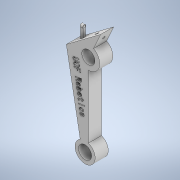
# Autodesk Inventor part: legV.1
Saved by Autodesk Inventor 2022 (Build 260153000, 153)
## iProperties
Created: 2022-01-23
Part Number: legV.1
Material: Generic
Document SubType Name: Modeling
Designer: money
Density: 1 g/cm^3
Appearance: Default
Author: money
Autodesk Inventor part; units mm, degrees
note: some values were not read from the file. Chosen so that the rebuilt part matches the saved one: sketch regions of "Extrusion1".
ref_plane "YZ Plane" through (0, 0, 0) normal (1, 0, 0) x (0, 1, 0)
ref_plane "XZ Plane" through (0, 0, 0) normal (0, 1, 0) x (-1, 0, 0)
ref_plane "XY Plane" through (0, 0, 0) normal (0, 0, 1) x (1, 0, 0)
sketch "Sketch1" plane through (0, 0, 0) normal (0, 0, 1) x (1, 0, 0)
  line L0 (25.584, 74.5203) -> (-8.8379, 48.7039)
  line L1 (25.584, 74.5203) -> (18.6122, 58.7142)
  arc A0 (13.3627, 37.1685) -> (18.6122, 58.7142) centre (13.3627, 48.5808) ccw
  circle A1 centre (13.3627, 48.5808) radius 6.604
  arc A2 (5.1377, -27.1634) -> (13.3627, -26.4893) centre (10.0086, -36.0797) ccw
  line L2 (-8.8379, 48.7039) -> (5.1377, -27.1634)
  line L3 (14.1717, -76.2055) -> (14.4802, -77.8797)
  line L4 (13.3627, 37.1685) -> (13.3627, -26.4893)
  circle A3 centre (10.0086, -36.0797) radius 6.604
  line L5 (3.7654, 42.7726) -> (3.9013, 41.8845)
  line L6 (3.9013, 41.8845) -> (-0.6634, 41.186)
  spline S0 degree 2 poles (-0.6634, 41.186) (-1.1355, 41.1137) (-1.3021, 40.8917) knots 0 0 0 1 1 1
  spline S1 degree 2 poles (-1.3021, 40.8917) (-1.4682, 40.6657) (-1.4063, 40.2616) knots 0 0 0 1 1 1
  line L7 (-1.4063, 40.2616) -> (-1.4014, 40.2296)
  spline S2 degree 2 poles (-1.4014, 40.2296) (-1.3439, 39.8536) (-1.1179, 39.6875) knots 0 0 0 1 1 1
  spline S3 degree 2 poles (-1.1179, 39.6875) (-0.8549, 39.4944) (-0.4149, 39.5617) knots 0 0 0 1 1 1
  line L8 (-0.4149, 39.5617) -> (4.1498, 40.2602)
  line L9 (4.1498, 40.2602) -> (4.2851, 39.3761)
  line L10 (4.2851, 39.3761) -> (-0.2796, 38.6776)
  spline S4 degree 2 poles (-0.2796, 38.6776) (-1.1317, 38.5472) (-1.6997, 38.968) knots 0 0 0 1 1 1
  spline S5 degree 2 poles (-1.6997, 38.968) (-2.1241, 39.2797) (-2.2496, 40.0998) knots 0 0 0 1 1 1
  line L11 (-2.2496, 40.0998) -> (-2.2545, 40.1318)
  spline S6 degree 2 poles (-2.2545, 40.1318) (-2.38, 40.952) (-2.0682, 41.3763) knots 0 0 0 1 1 1
  spline S7 degree 2 poles (-2.0682, 41.3763) (-1.6514, 41.9437) (-0.7993, 42.0741) knots 0 0 0 1 1 1
  line L12 (-0.7993, 42.0741) -> (3.7654, 42.7726)
  spline S8 degree 2 poles (1.1719, 34.5434) (-0.371, 34.4056) (-0.9753, 34.8495) knots 0 0 0 1 1 1
  spline S9 degree 2 poles (-0.9753, 34.8495) (-1.5058, 35.2391) (-1.6031, 35.8752) knots 0 0 0 1 1 1
  spline S10 degree 2 poles (-1.6031, 35.8752) (-1.6992, 36.5033) (-1.3102, 37.0378) knots 0 0 0 1 1 1
  spline S11 degree 2 poles (-1.3102, 37.0378) (-0.6257, 37.9696) (1.0706, 38.2291) knots 0 0 0 1 1 1
  spline S12 degree 2 poles (1.0706, 38.2291) (3.0509, 38.5321) (4.0524, 37.7929) knots 0 0 0 1 1 1
  spline S13 degree 2 poles (4.0524, 37.7929) (4.5875, 37.3998) (4.6787, 36.8037) knots 0 0 0 1 1 1
  spline S14 degree 2 poles (4.6787, 36.8037) (4.7755, 36.1716) (4.4637, 35.7472) knots 0 0 0 1 1 1
  spline S15 degree 2 poles (4.4637, 35.7472) (3.8843, 34.9585) (2.6392, 34.8007) knots 0 0 0 1 1 1
  line L13 (2.6392, 34.8007) -> (2.5088, 35.6528)
  spline S16 degree 2 poles (2.5088, 35.6528) (3.5521, 35.8452) (3.8265, 36.2188) knots 0 0 0 1 1 1
  spline S17 degree 2 poles (3.8265, 36.2188) (3.9655, 36.408) (3.9226, 36.688) knots 0 0 0 1 1 1
  spline S18 degree 2 poles (3.9226, 36.688) (3.8853, 36.9321) (3.6586, 37.1021) knots 0 0 0 1 1 1
  spline S19 degree 2 poles (3.6586, 37.1021) (2.9627, 37.6097) (1.2705, 37.3508) knots 0 0 0 1 1 1
  spline S20 degree 2 poles (1.2705, 37.3508) (-0.2057, 37.1249) (-0.6361, 36.5391) knots 0 0 0 1 1 1
  spline S21 degree 2 poles (-0.6361, 36.5391) (-0.8292, 36.2761) (-0.787, 36.0001) knots 0 0 0 1 1 1
  spline S22 degree 2 poles (-0.787, 36.0001) (-0.7484, 35.7481) (-0.4861, 35.5589) knots 0 0 0 1 1 1
  spline S23 degree 2 poles (-0.4861, 35.5589) (-0.1494, 35.3116) (1.0323, 35.4555) knots 0 0 0 1 1 1
  line L14 (1.0323, 35.4555) -> (1.1719, 34.5434)
  line L15 (-1.2517, 33.5789) -> (5.0252, 34.5394)
  line L16 (5.0252, 34.5394) -> (5.5548, 31.0789)
  line L17 (5.5548, 31.0789) -> (4.7986, 30.9632)
  line L18 (4.7986, 30.9632) -> (4.4044, 33.5395)
  line L19 (4.4044, 33.5395) -> (2.5241, 33.2518)
  line L20 (2.5241, 33.2518) -> (2.8223, 31.3035)
  line L21 (2.8223, 31.3035) -> (2.0661, 31.1878)
  line L22 (2.0661, 31.1878) -> (1.768, 33.1361)
  line L23 (1.768, 33.1361) -> (-1.1164, 32.6947)
  line L24 (-1.1164, 32.6947) -> (-1.2517, 33.5789)
  spline S24 degree 2 poles (6.5275, 24.7219) (6.653, 23.9018) (6.2097, 23.2935) knots 0 0 0 1 1 1
  spline S25 degree 2 poles (6.2097, 23.2935) (5.8438, 22.7953) (5.0597, 22.6754) knots 0 0 0 1 1 1
  spline S26 degree 2 poles (5.0597, 22.6754) (4.3396, 22.5652) (3.814, 22.9228) knots 0 0 0 1 1 1
  spline S27 degree 2 poles (3.814, 22.9228) (3.432, 23.1714) (3.3227, 23.4045) knots 0 0 0 1 1 1
  line L25 (3.3227, 23.4045) -> (0.5469, 21.8251)
  line L26 (0.5469, 21.8251) -> (0.4104, 22.7173)
  line L27 (0.4104, 22.7173) -> (3.0713, 24.2176)
  line L28 (3.0713, 24.2176) -> (2.9587, 24.9537)
  line L29 (2.9587, 24.9537) -> (0.1343, 24.5215)
  line L30 (0.1343, 24.5215) -> (-0.0016, 25.4097)
  line L31 (-0.0016, 25.4097) -> (6.2753, 26.3702)
  line L32 (6.2753, 26.3702) -> (6.5275, 24.7219)
  spline S28 degree 2 poles (3.8409, 24.2453) (3.8936, 23.9012) (4.1888, 23.6844) knots 0 0 0 1 1 1
  spline S29 degree 2 poles (4.1888, 23.6844) (4.4517, 23.4912) (4.9238, 23.5635) knots 0 0 0 1 1 1
  spline S30 degree 2 poles (4.9238, 23.5635) (5.3558, 23.6296) (5.5767, 23.9254) knots 0 0 0 1 1 1
  spline S31 degree 2 poles (5.5767, 23.9254) (5.824, 24.2622) (5.7475, 24.7622) knots 0 0 0 1 1 1
  line L33 (5.7475, 24.7622) -> (5.6551, 25.3663)
  line L34 (5.6551, 25.3663) -> (3.7148, 25.0694)
  line L35 (3.7148, 25.0694) -> (3.8409, 24.2453)
  spline S32 degree 2 poles (4.6294, 21.4467) (5.2337, 21.0029) (5.3445, 20.2788) knots 0 0 0 1 1 1
  spline S33 degree 2 poles (5.3445, 20.2788) (5.451, 19.5826) (5.0072, 18.9784) knots 0 0 0 1 1 1
  spline S34 degree 2 poles (5.0072, 18.9784) (4.5599, 18.3695) (3.3677, 18.1871) knots 0 0 0 1 1 1
  spline S35 degree 2 poles (3.3677, 18.1871) (2.2075, 18.0095) (1.5986, 18.4568) knots 0 0 0 1 1 1
  spline S36 degree 2 poles (1.5986, 18.4568) (0.9944, 18.9007) (0.8879, 19.5968) knots 0 0 0 1 1 1
  spline S37 degree 2 poles (0.8879, 19.5968) (0.777, 20.3209) (1.2209, 20.9252) knots 0 0 0 1 1 1
  spline S38 degree 2 poles (1.2209, 20.9252) (1.6642, 21.5334) (2.8284, 21.7116) knots 0 0 0 1 1 1
  spline S39 degree 2 poles (2.8284, 21.7116) (4.0246, 21.8946) (4.6294, 21.4467) knots 0 0 0 1 1 1
  spline S40 degree 2 poles (4.6204, 20.1679) (4.5684, 20.508) (4.2685, 20.7282) knots 0 0 0 1 1 1
  spline S41 degree 2 poles (4.2685, 20.7282) (3.8995, 20.9993) (2.9594, 20.8555) knots 0 0 0 1 1 1
  spline S42 degree 2 poles (2.9594, 20.8555) (2.0512, 20.7165) (1.7802, 20.3475) knots 0 0 0 1 1 1
  spline S43 degree 2 poles (1.7802, 20.3475) (1.5599, 20.0476) (1.612, 19.7076) knots 0 0 0 1 1 1
  spline S44 degree 2 poles (1.612, 19.7076) (1.6597, 19.3955) (1.9595, 19.1753) knots 0 0 0 1 1 1
  spline S45 degree 2 poles (1.9595, 19.1753) (2.3286, 18.9042) (3.2367, 19.0432) knots 0 0 0 1 1 1
  spline S46 degree 2 poles (3.2367, 19.0432) (4.1728, 19.1864) (4.4479, 19.5561) knots 0 0 0 1 1 1
  spline S47 degree 2 poles (4.4479, 19.5561) (4.6682, 19.8559) (4.6204, 20.1679) knots 0 0 0 1 1 1
  spline S48 degree 2 poles (5.148, 16.961) (5.8936, 16.6902) (6.0008, 15.9901) knots 0 0 0 1 1 1
  spline S49 degree 2 poles (6.0008, 15.9901) (6.0828, 15.454) (5.744, 14.9928) knots 0 0 0 1 1 1
  spline S50 degree 2 poles (5.744, 14.9928) (5.2967, 14.3839) (4.0765, 14.1972) knots 0 0 0 1 1 1
  spline S51 degree 2 poles (4.0765, 14.1972) (2.7883, 14) (2.1794, 14.4473) knots 0 0 0 1 1 1
  spline S52 degree 2 poles (2.1794, 14.4473) (1.6121, 14.8641) (1.53, 15.4002) knots 0 0 0 1 1 1
  spline S53 degree 2 poles (1.53, 15.4002) (1.4327, 16.0363) (1.9115, 16.4657) knots 0 0 0 1 1 1
  line L36 (1.9115, 16.4657) -> (1.3794, 16.3843)
  line L37 (1.3794, 16.3843) -> (1.2582, 17.1764)
  line L38 (1.2582, 17.1764) -> (7.5352, 18.1369)
  line L39 (7.5352, 18.1369) -> (7.6564, 17.3448)
  line L40 (7.6564, 17.3448) -> (5.148, 16.961)
  spline S54 degree 2 poles (3.4997, 16.7088) (2.6196, 16.5741) (2.3756, 16.242) knots 0 0 0 1 1 1
  spline S55 degree 2 poles (2.3756, 16.242) (2.1554, 15.9421) (2.1976, 15.6661) knots 0 0 0 1 1 1
  spline S56 degree 2 poles (2.1976, 15.6661) (2.2503, 15.322) (2.4763, 15.156) knots 0 0 0 1 1 1
  spline S57 degree 2 poles (2.4763, 15.156) (2.9191, 14.8307) (3.8913, 14.9795) knots 0 0 0 1 1 1
  spline S58 degree 2 poles (3.8913, 14.9795) (4.8274, 15.1227) (5.1296, 15.5293) knots 0 0 0 1 1 1
  spline S59 degree 2 poles (5.1296, 15.5293) (5.2956, 15.7553) (5.2479, 16.0673) knots 0 0 0 1 1 1
  spline S60 degree 2 poles (5.2479, 16.0673) (5.2008, 16.3754) (4.864, 16.6227) knots 0 0 0 1 1 1
  spline S61 degree 2 poles (4.864, 16.6227) (4.5319, 16.8667) (3.4997, 16.7088) knots 0 0 0 1 1 1
  spline S62 degree 2 poles (5.8844, 13.2455) (6.4887, 12.8016) (6.5995, 12.0775) knots 0 0 0 1 1 1
  spline S63 degree 2 poles (6.5995, 12.0775) (6.706, 11.3814) (6.2621, 10.7772) knots 0 0 0 1 1 1
  spline S64 degree 2 poles (6.2621, 10.7772) (5.8148, 10.1683) (4.6227, 9.9858) knots 0 0 0 1 1 1
  spline S65 degree 2 poles (4.6227, 9.9858) (3.4625, 9.8083) (2.8536, 10.2556) knots 0 0 0 1 1 1
  spline S66 degree 2 poles (2.8536, 10.2556) (2.2493, 10.6995) (2.1428, 11.3956) knots 0 0 0 1 1 1
  spline S67 degree 2 poles (2.1428, 11.3956) (2.032, 12.1197) (2.4759, 12.7239) knots 0 0 0 1 1 1
  spline S68 degree 2 poles (2.4759, 12.7239) (2.9192, 13.3322) (4.0833, 13.5104) knots 0 0 0 1 1 1
  spline S69 degree 2 poles (4.0833, 13.5104) (5.2795, 13.6934) (5.8844, 13.2455) knots 0 0 0 1 1 1
  spline S70 degree 2 poles (5.8754, 11.9667) (5.8233, 12.3068) (5.5235, 12.527) knots 0 0 0 1 1 1
  spline S71 degree 2 poles (5.5235, 12.527) (5.1545, 12.7981) (4.2143, 12.6542) knots 0 0 0 1 1 1
  spline S72 degree 2 poles (4.2143, 12.6542) (3.3062, 12.5153) (3.0351, 12.1462) knots 0 0 0 1 1 1
  spline S73 degree 2 poles (3.0351, 12.1462) (2.8149, 11.8464) (2.8669, 11.5064) knots 0 0 0 1 1 1
  spline S74 degree 2 poles (2.8669, 11.5064) (2.9147, 11.1943) (3.2145, 10.9741) knots 0 0 0 1 1 1
  spline S75 degree 2 poles (3.2145, 10.9741) (3.5835, 10.703) (4.4917, 10.842) knots 0 0 0 1 1 1
  spline S76 degree 2 poles (4.4917, 10.842) (5.4278, 10.9852) (5.7029, 11.3548) knots 0 0 0 1 1 1
  spline S77 degree 2 poles (5.7029, 11.3548) (5.9231, 11.6547) (5.8754, 11.9667) knots 0 0 0 1 1 1
  line L41 (6.4487, 8.648) -> (6.2951, 9.6522)
  line L42 (6.2951, 9.6522) -> (6.9552, 9.7532)
  line L43 (6.9552, 9.7532) -> (7.1088, 8.749)
  line L44 (7.1088, 8.749) -> (8.489, 8.9602)
  line L45 (8.489, 8.9602) -> (8.6102, 8.1681)
  line L46 (8.6102, 8.1681) -> (7.23, 7.9569)
  line L47 (7.23, 7.9569) -> (7.4461, 6.5447)
  line L48 (7.4461, 6.5447) -> (6.786, 6.4437)
  line L49 (6.786, 6.4437) -> (6.5699, 7.8559)
  line L50 (6.5699, 7.8559) -> (3.7935, 7.4311)
  spline S78 degree 2 poles (3.7935, 7.4311) (3.5295, 7.3907) (3.5937, 6.9706) knots 0 0 0 1 1 1
  spline S79 degree 2 poles (3.5937, 6.9706) (3.6727, 6.4545) (4.0224, 5.8284) knots 0 0 0 1 1 1
  line L51 (4.0224, 5.8284) -> (3.2223, 5.7059)
  spline S80 degree 2 poles (3.2223, 5.7059) (2.8878, 6.5268) (2.8229, 6.9509) knots 0 0 0 1 1 1
  spline S81 degree 2 poles (2.8229, 6.9509) (2.6521, 8.0671) (3.5483, 8.2042) knots 0 0 0 1 1 1
  line L52 (3.5483, 8.2042) -> (6.4487, 8.648)
  line L53 (3.4541, 2.8263) -> (3.3329, 3.6184)
  line L54 (3.3329, 3.6184) -> (7.7896, 4.3004)
  line L55 (7.7896, 4.3004) -> (7.9108, 3.5083)
  line L56 (7.9108, 3.5083) -> (3.4541, 2.8263)
  line L57 (9.731, 3.7868) -> (8.7549, 3.6374)
  line L58 (8.7549, 3.6374) -> (8.6337, 4.4295)
  line L59 (8.6337, 4.4295) -> (9.6098, 4.5789)
  line L60 (9.6098, 4.5789) -> (9.731, 3.7868)
  spline S82 degree 2 poles (6.9635, -1.2182) (7.4932, -1.0675) (7.6666, -0.8363) knots 0 0 0 1 1 1
  spline S83 degree 2 poles (7.6666, -0.8363) (7.8056, -0.6472) (7.7676, -0.3991) knots 0 0 0 1 1 1
  spline S84 degree 2 poles (7.7676, -0.3991) (7.7205, -0.0911) (7.4206, 0.1292) knots 0 0 0 1 1 1
  spline S85 degree 2 poles (7.4206, 0.1292) (7.0147, 0.4274) (6.0146, 0.2743) knots 0 0 0 1 1 1
  spline S86 degree 2 poles (6.0146, 0.2743) (5.1984, 0.1494) (4.9274, -0.2196) knots 0 0 0 1 1 1
  spline S87 degree 2 poles (4.9274, -0.2196) (4.7065, -0.5154) (4.7543, -0.8275) knots 0 0 0 1 1 1
  spline S88 degree 2 poles (4.7543, -0.8275) (4.7971, -1.1075) (5.06, -1.3007) knots 0 0 0 1 1 1
  spline S89 degree 2 poles (5.06, -1.3007) (5.3922, -1.5446) (6.128, -1.4034) knots 0 0 0 1 1 1
  line L61 (6.128, -1.4034) -> (6.2627, -2.2835)
  spline S90 degree 2 poles (6.2627, -2.2835) (5.276, -2.4713) (4.6671, -2.024) knots 0 0 0 1 1 1
  spline S91 degree 2 poles (4.6671, -2.024) (4.1367, -1.6344) (4.0302, -0.9383) knots 0 0 0 1 1 1
  spline S92 degree 2 poles (4.0302, -0.9383) (3.9236, -0.2422) (4.3675, 0.3621) knots 0 0 0 1 1 1
  spline S93 degree 2 poles (4.3675, 0.3621) (4.8385, 1.0033) (5.8787, 1.1624) knots 0 0 0 1 1 1
  spline S94 degree 2 poles (5.8787, 1.1624) (7.0708, 1.3449) (7.7858, 0.8197) knots 0 0 0 1 1 1
  spline S95 degree 2 poles (7.7858, 0.8197) (8.3901, 0.3758) (8.4917, -0.2883) knots 0 0 0 1 1 1
  spline S96 degree 2 poles (8.4917, -0.2883) (8.5927, -0.9484) (8.2539, -1.4097) knots 0 0 0 1 1 1
  spline S97 degree 2 poles (8.2539, -1.4097) (7.8919, -1.9073) (7.0933, -2.0663) knots 0 0 0 1 1 1
  line L62 (7.0933, -2.0663) -> (6.9635, -1.2182)
  spline S98 degree 2 poles (7.7644, -5.194) (8.1469, -5.0986) (8.2892, -4.9049) knots 0 0 0 1 1 1
  spline S99 degree 2 poles (8.2892, -4.9049) (8.4282, -4.7158) (8.3853, -4.4357) knots 0 0 0 1 1 1
  spline S100 degree 2 poles (8.3853, -4.4357) (8.3284, -4.0637) (8.1761, -3.9518) knots 0 0 0 1 1 1
  spline S101 degree 2 poles (8.1761, -3.9518) (7.987, -3.8129) (7.799, -3.8417) knots 0 0 0 1 1 1
  spline S102 degree 2 poles (7.799, -3.8417) (7.675, -3.8607) (7.5632, -4.0129) knots 0 0 0 1 1 1
  spline S103 degree 2 poles (7.5632, -4.0129) (7.387, -4.2528) (7.2423, -5.02) knots 0 0 0 1 1 1
  spline S104 degree 2 poles (7.2423, -5.02) (7.1434, -5.6043) (6.9198, -5.9087) knots 0 0 0 1 1 1
  spline S105 degree 2 poles (6.9198, -5.9087) (6.6589, -6.2639) (6.1588, -6.3404) knots 0 0 0 1 1 1
  spline S106 degree 2 poles (6.1588, -6.3404) (5.6867, -6.4127) (5.2946, -6.1247) knots 0 0 0 1 1 1
  spline S107 degree 2 poles (5.2946, -6.1247) (4.7642, -5.735) (4.6527, -5.0069) knots 0 0 0 1 1 1
  spline S108 degree 2 poles (4.6527, -5.0069) (4.5321, -4.2188) (4.867, -3.7581) knots 0 0 0 1 1 1
  spline S109 degree 2 poles (4.867, -3.7581) (5.2335, -3.2639) (6.2306, -3.1441) knots 0 0 0 1 1 1
  line L63 (6.2306, -3.1441) -> (6.3512, -3.9322)
  spline S110 degree 2 poles (6.3512, -3.9322) (5.6151, -4.0449) (5.4762, -4.234) knots 0 0 0 1 1 1
  spline S111 degree 2 poles (5.4762, -4.234) (5.3101, -4.46) (5.372, -4.8641) knots 0 0 0 1 1 1
  spline S112 degree 2 poles (5.372, -4.8641) (5.4344, -5.2721) (5.6604, -5.4382) knots 0 0 0 1 1 1
  spline S113 degree 2 poles (5.6604, -5.4382) (5.8495, -5.5771) (6.0696, -5.5434) knots 0 0 0 1 1 1
  spline S114 degree 2 poles (6.0696, -5.5434) (6.2216, -5.5202) (6.3605, -5.331) knots 0 0 0 1 1 1
  spline S115 degree 2 poles (6.3605, -5.331) (6.5096, -5.1281) (6.6147, -4.5838) knots 0 0 0 1 1 1
  spline S116 degree 2 poles (6.6147, -4.5838) (6.7797, -3.7356) (7.0033, -3.4312) knots 0 0 0 1 1 1
  spline S117 degree 2 poles (7.0033, -3.4312) (7.2608, -3.0806) (7.7049, -3.0127) knots 0 0 0 1 1 1
  spline S118 degree 2 poles (7.7049, -3.0127) (8.145, -2.9453) (8.5693, -3.2571) knots 0 0 0 1 1 1
  spline S119 degree 2 poles (8.5693, -3.2571) (8.9937, -3.5688) (9.1094, -4.3249) knots 0 0 0 1 1 1
  spline S120 degree 2 poles (9.1094, -4.3249) (9.211, -4.989) (8.8722, -5.4503) knots 0 0 0 1 1 1
  spline S121 degree 2 poles (8.8722, -5.4503) (8.5333, -5.9116) (7.8837, -5.9741) knots 0 0 0 1 1 1
  line L64 (7.8837, -5.9741) -> (7.7644, -5.194)
  point P0 (7.4727, 18.545)
  dimension "d2" = 152.4
  dimension "d3" = 10.16
  dimension "d4" = 13.208
  dimension "d5" = 13.208
  constraints: 10 end point, 4 centre point, 4 point on circle, 2 coincident, 1 other
  measures "d2" vertical distance of L3.end L0.start
  measures "d3" radius of A2
  measures "d4" diameter of A3
  measures "d5" diameter of A1
extrude "Extrusion1" add sketch "Sketch1" along normal blind 13.208 contours L1 A0 L4 A2 L2 L0 | L5 L6 S0 S1 L7 S2 S3 L8 L9 L10 S4 S5 L11 S6 S7 L12 | S8 S9 S10 S11 S12 S13 S14 S15 L13 S16 S17 S18 S19 S20 S21 S22 S23 L14 | L15 L16 L17 L18 L19 L20 L21 L22 L23 L24 | S24 S25 S26 S27 L25 L26 L27 L28 L29 L30 L31 L32 | S32 S33 S34 S35 S36 S37 S38 S39 | S48 S49 S50 S51 S52 S53 L36 L37 L38 L39 L40 | S62 S63 S64 S65 S66 S67 S68 S69 | L41 L42 L43 L44 L45 L46 L47 L48 L49 L50 S78 S79 L51 S80 S81 L52 | L53 L54 L55 L56 | L57 L58 L59 L60 | S82 S83 S84 S85 S86 S87 S88 S89 L61 S90 S91 S92 S93 S94 S95 S96 S97 L62 | S98 S99 S100 S101 S102 S103 S104 S105 S106 S107 S108 S109 L63 S110 S111 S112 S113 S114 S115 S116 S117 S118 S119 S120 S121 L64
sketch "Sketch2" plane through (0, 0, 13.208) normal (0, 0, 1) x (1, 0, 0)
  line L0 (3.7654, 42.7726) -> (3.9013, 41.8845)
  line L1 (3.9013, 41.8845) -> (-0.6634, 41.186)
  spline S0 degree 2 poles (-0.6634, 41.186) (-1.1355, 41.1137) (-1.3021, 40.8917) knots 0 0 0 1 1 1
  spline S1 degree 2 poles (-1.3021, 40.8917) (-1.4682, 40.6657) (-1.4063, 40.2616) knots 0 0 0 1 1 1
  line L2 (-1.4063, 40.2616) -> (-1.4014, 40.2296)
  spline S2 degree 2 poles (-1.4014, 40.2296) (-1.3439, 39.8536) (-1.1179, 39.6875) knots 0 0 0 1 1 1
  spline S3 degree 2 poles (-1.1179, 39.6875) (-0.8549, 39.4944) (-0.4149, 39.5617) knots 0 0 0 1 1 1
  line L3 (-0.4149, 39.5617) -> (4.1498, 40.2602)
  line L4 (4.1498, 40.2602) -> (4.2851, 39.3761)
  line L5 (4.2851, 39.3761) -> (-0.2796, 38.6776)
  spline S4 degree 2 poles (-0.2796, 38.6776) (-1.1317, 38.5472) (-1.6997, 38.968) knots 0 0 0 1 1 1
  spline S5 degree 2 poles (-1.6997, 38.968) (-2.1241, 39.2797) (-2.2496, 40.0998) knots 0 0 0 1 1 1
  line L6 (-2.2496, 40.0998) -> (-2.2545, 40.1318)
  spline S6 degree 2 poles (-2.2545, 40.1318) (-2.38, 40.952) (-2.0682, 41.3763) knots 0 0 0 1 1 1
  spline S7 degree 2 poles (-2.0682, 41.3763) (-1.6514, 41.9437) (-0.7993, 42.0741) knots 0 0 0 1 1 1
  line L7 (-0.7993, 42.0741) -> (3.7654, 42.7726)
  spline S8 degree 2 poles (1.1719, 34.5434) (-0.371, 34.4056) (-0.9753, 34.8495) knots 0 0 0 1 1 1
  spline S9 degree 2 poles (-0.9753, 34.8495) (-1.5058, 35.2391) (-1.6031, 35.8752) knots 0 0 0 1 1 1
  spline S10 degree 2 poles (-1.6031, 35.8752) (-1.6992, 36.5033) (-1.3102, 37.0378) knots 0 0 0 1 1 1
  spline S11 degree 2 poles (-1.3102, 37.0378) (-0.6257, 37.9696) (1.0706, 38.2291) knots 0 0 0 1 1 1
  spline S12 degree 2 poles (1.0706, 38.2291) (3.0509, 38.5321) (4.0524, 37.7929) knots 0 0 0 1 1 1
  spline S13 degree 2 poles (4.0524, 37.7929) (4.5875, 37.3998) (4.6787, 36.8037) knots 0 0 0 1 1 1
  spline S14 degree 2 poles (4.6787, 36.8037) (4.7755, 36.1716) (4.4637, 35.7472) knots 0 0 0 1 1 1
  spline S15 degree 2 poles (4.4637, 35.7472) (3.8843, 34.9585) (2.6392, 34.8007) knots 0 0 0 1 1 1
  line L8 (2.6392, 34.8007) -> (2.5088, 35.6528)
  spline S16 degree 2 poles (2.5088, 35.6528) (3.5521, 35.8452) (3.8265, 36.2188) knots 0 0 0 1 1 1
  spline S17 degree 2 poles (3.8265, 36.2188) (3.9655, 36.408) (3.9226, 36.688) knots 0 0 0 1 1 1
  spline S18 degree 2 poles (3.9226, 36.688) (3.8853, 36.9321) (3.6586, 37.1021) knots 0 0 0 1 1 1
  spline S19 degree 2 poles (3.6586, 37.1021) (2.9627, 37.6097) (1.2705, 37.3508) knots 0 0 0 1 1 1
  spline S20 degree 2 poles (1.2705, 37.3508) (-0.2057, 37.1249) (-0.6361, 36.5391) knots 0 0 0 1 1 1
  spline S21 degree 2 poles (-0.6361, 36.5391) (-0.8292, 36.2761) (-0.787, 36.0001) knots 0 0 0 1 1 1
  spline S22 degree 2 poles (-0.787, 36.0001) (-0.7484, 35.7481) (-0.4861, 35.5589) knots 0 0 0 1 1 1
  spline S23 degree 2 poles (-0.4861, 35.5589) (-0.1494, 35.3116) (1.0323, 35.4555) knots 0 0 0 1 1 1
  line L9 (1.0323, 35.4555) -> (1.1719, 34.5434)
  line L10 (-1.2517, 33.5789) -> (5.0252, 34.5394)
  line L11 (5.0252, 34.5394) -> (5.5548, 31.0789)
  line L12 (5.5548, 31.0789) -> (4.7986, 30.9632)
  line L13 (4.7986, 30.9632) -> (4.4044, 33.5395)
  line L14 (4.4044, 33.5395) -> (2.5241, 33.2518)
  line L15 (2.5241, 33.2518) -> (2.8223, 31.3035)
  line L16 (2.8223, 31.3035) -> (2.0661, 31.1878)
  line L17 (2.0661, 31.1878) -> (1.768, 33.1361)
  line L18 (1.768, 33.1361) -> (-1.1164, 32.6947)
  line L19 (-1.1164, 32.6947) -> (-1.2517, 33.5789)
  spline S24 degree 2 poles (6.5275, 24.7219) (6.653, 23.9018) (6.2097, 23.2935) knots 0 0 0 1 1 1
  spline S25 degree 2 poles (6.2097, 23.2935) (5.8438, 22.7953) (5.0597, 22.6754) knots 0 0 0 1 1 1
  spline S26 degree 2 poles (5.0597, 22.6754) (4.3396, 22.5652) (3.814, 22.9228) knots 0 0 0 1 1 1
  spline S27 degree 2 poles (3.814, 22.9228) (3.432, 23.1714) (3.3227, 23.4045) knots 0 0 0 1 1 1
  line L20 (3.3227, 23.4045) -> (0.5469, 21.8251)
  line L21 (0.5469, 21.8251) -> (0.4104, 22.7173)
  line L22 (0.4104, 22.7173) -> (3.0713, 24.2176)
  line L23 (3.0713, 24.2176) -> (2.9587, 24.9537)
  line L24 (2.9587, 24.9537) -> (0.1343, 24.5215)
  line L25 (0.1343, 24.5215) -> (-0.0016, 25.4097)
  line L26 (-0.0016, 25.4097) -> (6.2753, 26.3702)
  line L27 (6.2753, 26.3702) -> (6.5275, 24.7219)
  spline S28 degree 2 poles (3.8409, 24.2453) (3.8936, 23.9012) (4.1888, 23.6844) knots 0 0 0 1 1 1
  spline S29 degree 2 poles (4.1888, 23.6844) (4.4517, 23.4912) (4.9238, 23.5635) knots 0 0 0 1 1 1
  spline S30 degree 2 poles (4.9238, 23.5635) (5.3558, 23.6296) (5.5767, 23.9254) knots 0 0 0 1 1 1
  spline S31 degree 2 poles (5.5767, 23.9254) (5.824, 24.2622) (5.7475, 24.7622) knots 0 0 0 1 1 1
  line L28 (5.7475, 24.7622) -> (5.6551, 25.3663)
  line L29 (5.6551, 25.3663) -> (3.7148, 25.0694)
  line L30 (3.7148, 25.0694) -> (3.8409, 24.2453)
  spline S32 degree 2 poles (4.6294, 21.4467) (5.2337, 21.0029) (5.3445, 20.2788) knots 0 0 0 1 1 1
  spline S33 degree 2 poles (5.3445, 20.2788) (5.451, 19.5826) (5.0072, 18.9784) knots 0 0 0 1 1 1
  spline S34 degree 2 poles (5.0072, 18.9784) (4.5599, 18.3695) (3.3677, 18.1871) knots 0 0 0 1 1 1
  spline S35 degree 2 poles (3.3677, 18.1871) (2.2075, 18.0095) (1.5986, 18.4568) knots 0 0 0 1 1 1
  spline S36 degree 2 poles (1.5986, 18.4568) (0.9944, 18.9007) (0.8879, 19.5968) knots 0 0 0 1 1 1
  spline S37 degree 2 poles (0.8879, 19.5968) (0.777, 20.3209) (1.2209, 20.9252) knots 0 0 0 1 1 1
  spline S38 degree 2 poles (1.2209, 20.9252) (1.6642, 21.5334) (2.8284, 21.7116) knots 0 0 0 1 1 1
  spline S39 degree 2 poles (2.8284, 21.7116) (4.0246, 21.8946) (4.6294, 21.4467) knots 0 0 0 1 1 1
  spline S40 degree 2 poles (4.6204, 20.1679) (4.5684, 20.508) (4.2685, 20.7282) knots 0 0 0 1 1 1
  spline S41 degree 2 poles (4.2685, 20.7282) (3.8995, 20.9993) (2.9594, 20.8555) knots 0 0 0 1 1 1
  spline S42 degree 2 poles (2.9594, 20.8555) (2.0512, 20.7165) (1.7802, 20.3475) knots 0 0 0 1 1 1
  spline S43 degree 2 poles (1.7802, 20.3475) (1.5599, 20.0476) (1.612, 19.7076) knots 0 0 0 1 1 1
  spline S44 degree 2 poles (1.612, 19.7076) (1.6597, 19.3955) (1.9595, 19.1753) knots 0 0 0 1 1 1
  spline S45 degree 2 poles (1.9595, 19.1753) (2.3286, 18.9042) (3.2367, 19.0432) knots 0 0 0 1 1 1
  spline S46 degree 2 poles (3.2367, 19.0432) (4.1728, 19.1864) (4.4479, 19.5561) knots 0 0 0 1 1 1
  spline S47 degree 2 poles (4.4479, 19.5561) (4.6682, 19.8559) (4.6204, 20.1679) knots 0 0 0 1 1 1
  spline S48 degree 2 poles (5.148, 16.961) (5.8936, 16.6902) (6.0008, 15.9901) knots 0 0 0 1 1 1
  spline S49 degree 2 poles (6.0008, 15.9901) (6.0828, 15.454) (5.744, 14.9928) knots 0 0 0 1 1 1
  spline S50 degree 2 poles (5.744, 14.9928) (5.2967, 14.3839) (4.0765, 14.1972) knots 0 0 0 1 1 1
  spline S51 degree 2 poles (4.0765, 14.1972) (2.7883, 14) (2.1794, 14.4473) knots 0 0 0 1 1 1
  spline S52 degree 2 poles (2.1794, 14.4473) (1.6121, 14.8641) (1.53, 15.4002) knots 0 0 0 1 1 1
  spline S53 degree 2 poles (1.53, 15.4002) (1.4327, 16.0363) (1.9115, 16.4657) knots 0 0 0 1 1 1
  line L31 (1.9115, 16.4657) -> (1.3794, 16.3843)
  line L32 (1.3794, 16.3843) -> (1.2582, 17.1764)
  line L33 (1.2582, 17.1764) -> (7.5352, 18.1369)
  line L34 (7.5352, 18.1369) -> (7.6564, 17.3448)
  line L35 (7.6564, 17.3448) -> (5.148, 16.961)
  spline S54 degree 2 poles (3.4997, 16.7088) (2.6196, 16.5741) (2.3756, 16.242) knots 0 0 0 1 1 1
  spline S55 degree 2 poles (2.3756, 16.242) (2.1554, 15.9421) (2.1976, 15.6661) knots 0 0 0 1 1 1
  spline S56 degree 2 poles (2.1976, 15.6661) (2.2503, 15.322) (2.4763, 15.156) knots 0 0 0 1 1 1
  spline S57 degree 2 poles (2.4763, 15.156) (2.9191, 14.8307) (3.8913, 14.9795) knots 0 0 0 1 1 1
  spline S58 degree 2 poles (3.8913, 14.9795) (4.8274, 15.1227) (5.1296, 15.5293) knots 0 0 0 1 1 1
  spline S59 degree 2 poles (5.1296, 15.5293) (5.2956, 15.7553) (5.2479, 16.0673) knots 0 0 0 1 1 1
  spline S60 degree 2 poles (5.2479, 16.0673) (5.2008, 16.3754) (4.864, 16.6227) knots 0 0 0 1 1 1
  spline S61 degree 2 poles (4.864, 16.6227) (4.5319, 16.8667) (3.4997, 16.7088) knots 0 0 0 1 1 1
  spline S62 degree 2 poles (5.8844, 13.2455) (6.4887, 12.8016) (6.5995, 12.0775) knots 0 0 0 1 1 1
  spline S63 degree 2 poles (6.5995, 12.0775) (6.706, 11.3814) (6.2621, 10.7772) knots 0 0 0 1 1 1
  spline S64 degree 2 poles (6.2621, 10.7772) (5.8148, 10.1683) (4.6227, 9.9858) knots 0 0 0 1 1 1
  spline S65 degree 2 poles (4.6227, 9.9858) (3.4625, 9.8083) (2.8536, 10.2556) knots 0 0 0 1 1 1
  spline S66 degree 2 poles (2.8536, 10.2556) (2.2493, 10.6995) (2.1428, 11.3956) knots 0 0 0 1 1 1
  spline S67 degree 2 poles (2.1428, 11.3956) (2.032, 12.1197) (2.4759, 12.7239) knots 0 0 0 1 1 1
  spline S68 degree 2 poles (2.4759, 12.7239) (2.9192, 13.3322) (4.0833, 13.5104) knots 0 0 0 1 1 1
  spline S69 degree 2 poles (4.0833, 13.5104) (5.2795, 13.6934) (5.8844, 13.2455) knots 0 0 0 1 1 1
  spline S70 degree 2 poles (5.8754, 11.9667) (5.8233, 12.3068) (5.5235, 12.527) knots 0 0 0 1 1 1
  spline S71 degree 2 poles (5.5235, 12.527) (5.1545, 12.7981) (4.2143, 12.6542) knots 0 0 0 1 1 1
  spline S72 degree 2 poles (4.2143, 12.6542) (3.3062, 12.5153) (3.0351, 12.1462) knots 0 0 0 1 1 1
  spline S73 degree 2 poles (3.0351, 12.1462) (2.8149, 11.8464) (2.8669, 11.5064) knots 0 0 0 1 1 1
  spline S74 degree 2 poles (2.8669, 11.5064) (2.9147, 11.1943) (3.2145, 10.9741) knots 0 0 0 1 1 1
  spline S75 degree 2 poles (3.2145, 10.9741) (3.5835, 10.703) (4.4917, 10.842) knots 0 0 0 1 1 1
  spline S76 degree 2 poles (4.4917, 10.842) (5.4278, 10.9852) (5.7029, 11.3548) knots 0 0 0 1 1 1
  spline S77 degree 2 poles (5.7029, 11.3548) (5.9231, 11.6547) (5.8754, 11.9667) knots 0 0 0 1 1 1
  line L36 (6.4487, 8.648) -> (6.2951, 9.6522)
  line L37 (6.2951, 9.6522) -> (6.9552, 9.7532)
  line L38 (6.9552, 9.7532) -> (7.1088, 8.749)
  line L39 (7.1088, 8.749) -> (8.489, 8.9602)
  line L40 (8.489, 8.9602) -> (8.6102, 8.1681)
  line L41 (8.6102, 8.1681) -> (7.23, 7.9569)
  line L42 (7.23, 7.9569) -> (7.4461, 6.5447)
  line L43 (7.4461, 6.5447) -> (6.786, 6.4437)
  line L44 (6.786, 6.4437) -> (6.5699, 7.8559)
  line L45 (6.5699, 7.8559) -> (3.7935, 7.4311)
  spline S78 degree 2 poles (3.7935, 7.4311) (3.5295, 7.3907) (3.5937, 6.9706) knots 0 0 0 1 1 1
  spline S79 degree 2 poles (3.5937, 6.9706) (3.6727, 6.4545) (4.0224, 5.8284) knots 0 0 0 1 1 1
  line L46 (4.0224, 5.8284) -> (3.2223, 5.7059)
  spline S80 degree 2 poles (3.2223, 5.7059) (2.8878, 6.5268) (2.8229, 6.9509) knots 0 0 0 1 1 1
  spline S81 degree 2 poles (2.8229, 6.9509) (2.6521, 8.0671) (3.5483, 8.2042) knots 0 0 0 1 1 1
  line L47 (3.5483, 8.2042) -> (6.4487, 8.648)
  line L48 (3.4541, 2.8263) -> (3.3329, 3.6184)
  line L49 (3.3329, 3.6184) -> (7.7896, 4.3004)
  line L50 (7.7896, 4.3004) -> (7.9108, 3.5083)
  line L51 (7.9108, 3.5083) -> (3.4541, 2.8263)
  line L52 (9.731, 3.7868) -> (8.7549, 3.6374)
  line L53 (8.7549, 3.6374) -> (8.6337, 4.4295)
  line L54 (8.6337, 4.4295) -> (9.6098, 4.5789)
  line L55 (9.6098, 4.5789) -> (9.731, 3.7868)
  spline S82 degree 2 poles (6.9635, -1.2182) (7.4932, -1.0675) (7.6666, -0.8363) knots 0 0 0 1 1 1
  spline S83 degree 2 poles (7.6666, -0.8363) (7.8056, -0.6472) (7.7676, -0.3991) knots 0 0 0 1 1 1
  spline S84 degree 2 poles (7.7676, -0.3991) (7.7205, -0.0911) (7.4206, 0.1292) knots 0 0 0 1 1 1
  spline S85 degree 2 poles (7.4206, 0.1292) (7.0147, 0.4274) (6.0146, 0.2743) knots 0 0 0 1 1 1
  spline S86 degree 2 poles (6.0146, 0.2743) (5.1984, 0.1494) (4.9274, -0.2196) knots 0 0 0 1 1 1
  spline S87 degree 2 poles (4.9274, -0.2196) (4.7065, -0.5154) (4.7543, -0.8275) knots 0 0 0 1 1 1
  spline S88 degree 2 poles (4.7543, -0.8275) (4.7971, -1.1075) (5.06, -1.3007) knots 0 0 0 1 1 1
  spline S89 degree 2 poles (5.06, -1.3007) (5.3922, -1.5446) (6.128, -1.4034) knots 0 0 0 1 1 1
  line L56 (6.128, -1.4034) -> (6.2627, -2.2835)
  spline S90 degree 2 poles (6.2627, -2.2835) (5.276, -2.4713) (4.6671, -2.024) knots 0 0 0 1 1 1
  spline S91 degree 2 poles (4.6671, -2.024) (4.1367, -1.6344) (4.0302, -0.9383) knots 0 0 0 1 1 1
  spline S92 degree 2 poles (4.0302, -0.9383) (3.9236, -0.2422) (4.3675, 0.3621) knots 0 0 0 1 1 1
  spline S93 degree 2 poles (4.3675, 0.3621) (4.8385, 1.0033) (5.8787, 1.1624) knots 0 0 0 1 1 1
  spline S94 degree 2 poles (5.8787, 1.1624) (7.0708, 1.3449) (7.7858, 0.8197) knots 0 0 0 1 1 1
  spline S95 degree 2 poles (7.7858, 0.8197) (8.3901, 0.3758) (8.4917, -0.2883) knots 0 0 0 1 1 1
  spline S96 degree 2 poles (8.4917, -0.2883) (8.5927, -0.9484) (8.2539, -1.4097) knots 0 0 0 1 1 1
  spline S97 degree 2 poles (8.2539, -1.4097) (7.8919, -1.9073) (7.0933, -2.0663) knots 0 0 0 1 1 1
  line L57 (7.0933, -2.0663) -> (6.9635, -1.2182)
  spline S98 degree 2 poles (7.7644, -5.194) (8.1469, -5.0986) (8.2892, -4.9049) knots 0 0 0 1 1 1
  spline S99 degree 2 poles (8.2892, -4.9049) (8.4282, -4.7158) (8.3853, -4.4357) knots 0 0 0 1 1 1
  spline S100 degree 2 poles (8.3853, -4.4357) (8.3284, -4.0637) (8.1761, -3.9518) knots 0 0 0 1 1 1
  spline S101 degree 2 poles (8.1761, -3.9518) (7.987, -3.8129) (7.799, -3.8417) knots 0 0 0 1 1 1
  spline S102 degree 2 poles (7.799, -3.8417) (7.675, -3.8607) (7.5632, -4.0129) knots 0 0 0 1 1 1
  spline S103 degree 2 poles (7.5632, -4.0129) (7.387, -4.2528) (7.2423, -5.02) knots 0 0 0 1 1 1
  spline S104 degree 2 poles (7.2423, -5.02) (7.1434, -5.6043) (6.9198, -5.9087) knots 0 0 0 1 1 1
  spline S105 degree 2 poles (6.9198, -5.9087) (6.6589, -6.2639) (6.1588, -6.3404) knots 0 0 0 1 1 1
  spline S106 degree 2 poles (6.1588, -6.3404) (5.6867, -6.4127) (5.2946, -6.1247) knots 0 0 0 1 1 1
  spline S107 degree 2 poles (5.2946, -6.1247) (4.7642, -5.735) (4.6527, -5.0069) knots 0 0 0 1 1 1
  spline S108 degree 2 poles (4.6527, -5.0069) (4.5321, -4.2188) (4.867, -3.7581) knots 0 0 0 1 1 1
  spline S109 degree 2 poles (4.867, -3.7581) (5.2335, -3.2639) (6.2306, -3.1441) knots 0 0 0 1 1 1
  line L58 (6.2306, -3.1441) -> (6.3512, -3.9322)
  spline S110 degree 2 poles (6.3512, -3.9322) (5.6151, -4.0449) (5.4762, -4.234) knots 0 0 0 1 1 1
  spline S111 degree 2 poles (5.4762, -4.234) (5.3101, -4.46) (5.372, -4.8641) knots 0 0 0 1 1 1
  spline S112 degree 2 poles (5.372, -4.8641) (5.4344, -5.2721) (5.6604, -5.4382) knots 0 0 0 1 1 1
  spline S113 degree 2 poles (5.6604, -5.4382) (5.8495, -5.5771) (6.0696, -5.5434) knots 0 0 0 1 1 1
  spline S114 degree 2 poles (6.0696, -5.5434) (6.2216, -5.5202) (6.3605, -5.331) knots 0 0 0 1 1 1
  spline S115 degree 2 poles (6.3605, -5.331) (6.5096, -5.1281) (6.6147, -4.5838) knots 0 0 0 1 1 1
  spline S116 degree 2 poles (6.6147, -4.5838) (6.7797, -3.7356) (7.0033, -3.4312) knots 0 0 0 1 1 1
  spline S117 degree 2 poles (7.0033, -3.4312) (7.2608, -3.0806) (7.7049, -3.0127) knots 0 0 0 1 1 1
  spline S118 degree 2 poles (7.7049, -3.0127) (8.145, -2.9453) (8.5693, -3.2571) knots 0 0 0 1 1 1
  spline S119 degree 2 poles (8.5693, -3.2571) (8.9937, -3.5688) (9.1094, -4.3249) knots 0 0 0 1 1 1
  spline S120 degree 2 poles (9.1094, -4.3249) (9.211, -4.989) (8.8722, -5.4503) knots 0 0 0 1 1 1
  spline S121 degree 2 poles (8.8722, -5.4503) (8.5333, -5.9116) (7.8837, -5.9741) knots 0 0 0 1 1 1
  line L59 (7.8837, -5.9741) -> (7.7644, -5.194)
  point P0 (0, 0)
  point P1 (7.4727, 18.545)
  constraints: 1 other
extrude "Extrusion2" cut sketch "Sketch2" against normal blind 34.417
sketch "Sketch3" plane through (0, 0, 0) normal (1, 0, 0) x (0, 1, 0)
  line L0 (74.5203, 13.208) -> (48.7039, 13.208) projected
  line L1 (66.7838, 13.208) -> (67.1094, 0)
  line L2 (74.5203, 0) -> (48.7039, 0) projected
  line L3 (66.7838, 13.208) -> (66.7838, 0)
  circle A0 centre (66.7838, 6.604) radius 1.27
  point P0 (0, 0)
  dimension "d10" = 2.54
  constraints: 4 end point, 3 point on line, 1 centre point, 1 midpoint, 1 perpendicular
  measures "d10" diameter of A0
extrude "Extrusion3" cut sketch "Sketch3" along normal blind 105.283 contours A0 L1 | L1 A0 L3 | L3 A0 picked at (66.8923, 6.1833)
sketch "Sketch4" plane through (0, 0, 0) normal (1, 0, 0) x (0, 1, 0)
  circle A0 centre (66.7838, 6.604) radius 1.27 projected
  circle A1 centre (66.7838, 6.604) radius 1.27
  line L0 (65.7449, 5.334) -> (51.2377, 5.334)
  line L1 (51.2377, 5.334) -> (51.2377, 7.874)
  line L2 (55.1848, 13.208) -> (55.1848, 0) projected
  line L3 (51.2377, 7.874) -> (65.7449, 7.874)
  arc A2 (65.7449, 5.334) -> (65.7449, 7.874) centre (66.7838, 6.604) ccw
  point P0 (0, 0)
  constraints: 6 end point, 2 centre point, 2 coincident, 2 point on circle, 1 horizontal, 1 parallel, 1 tangent
extrude "Extrusion4" add sketch "Sketch4" along normal blind 2.667
equation "\"d6\" = d5"
body "Solid1"
